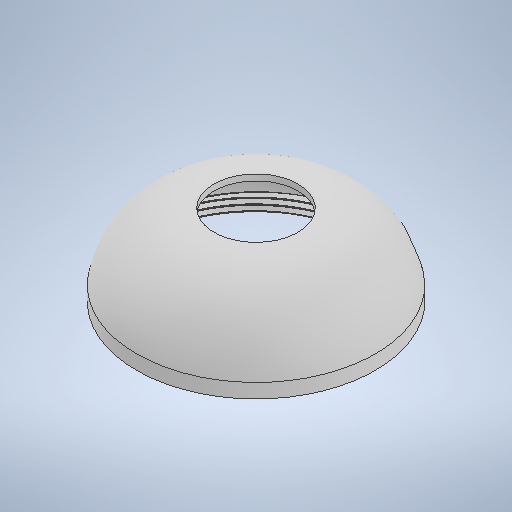
# Autodesk Inventor part: Cylinder Housing_cap
Saved by Autodesk Inventor 2025 (Build 290162000, 162)
## iProperties
Created: 2025-07-15
Part Number: Cylinder Housing_cap
Material: Generic
Document SubType Name: Modeling
Designer: mumin
Density: 1 g/cm^3
Appearance: Default
Author: mumin
Autodesk Inventor part; units mm, degrees
ref_plane "YZ Plane" through (0, 0, 0) normal (1, 0, 0) x (0, 1, 0)
ref_plane "XZ Plane" through (0, 0, 0) normal (0, 1, 0) x (-1, 0, 0)
ref_plane "XY Plane" through (0, 0, 0) normal (0, 0, 1) x (1, 0, 0)
sketch "Sketch1" plane through (0, 0, 0) normal (1, 0, 0) x (0, 1, 0)
  line L0 (-19.2867, 0) -> (115.7202, 0) projected
  line L1 (0, -116) -> (0, -121)
  line L2 (0, -116) -> (14.5, -116)
  line L3 (0, -121) -> (14.5, -121)
  line L4 (75.884, 0) -> (75.884, -42.5)
  arc A0 (14.5, -116) -> (75.884, -42.5) centre (1.1882, -42.5) ccw
  line L5 (75.884, -42.5) -> (82.0374, -42.5)
  arc A1 (14.5, -121) -> (82.0374, -42.5) centre (1.9607, -41.909) ccw
  point P0 (0, 0)
  dimension "d0" = 116
  dimension "d1" = 14.5
  dimension "d2" = 5
  dimension "d3" = 42.5
  constraints: 10 end point, 4 point on circle, 3 horizontal, 2 centre point, 2 vertical, 1 point on line, 1 tangent
  measures "d0" distance from line of L0 L1.start
  measures "d1" distance of L1.start L2.end
  measures "d2" distance of L1.start L1.end
  measures "d3" distance of L4.start L4.end
revolve "Revolution1" add sketch "Sketch1" angle 360 about axis through (0, -10, 0) along (0, 1, 0)
sketch "Sketch4" plane through (0, 0, 0) normal (0, 0, 1) x (1, 0, 0)
  arc A0 (74.226, 20) -> (32.226, 20) centre (53.226, 20) ccw
  line L0 (0, -8.9518) -> (0, 53.7108) projected
  line L1 (121, 0) -> (-121, 0) construction
  line L2 (32.226, 20) -> (32.226, 0)
  line L3 (32.226, 0) -> (74.226, 0)
  line L4 (74.226, 0) -> (74.226, 20)
  point P0 (0, 0)
  dimension "d26" = 42
  dimension "d27" = 53.226
  dimension "d28" = 20
  constraints: 6 end point, 2 point on circle, 1 centre point, 1 parallel, 1 point on line
  measures "d26" diameter of A0
  measures "d27" distance from line of L0 A0.centre
  measures "d28" distance from line of L1 A0.centre
extrude "LV Hole" cut sketch "Sketch4" against normal through all
thread "Thread2" size "M235x6" class "6H" standard "ANSI Metric M Profile" length 14.5
sketch "Sketch8" plane through (0, 14.5, 0) normal (1, 0, 0) x (0, 0, 1)
  line L0 (116, 0) -> (116, 14.5)
  line L1 (116, 14.5) -> (111.5512, 14.5)
  line L2 (111.5512, 14.5) -> (111.5512, 0)
  line L3 (111.5512, 0) -> (116, 0)
  line L4 (0, -83.9448) -> (0, 30.9075) projected
  constraints: 8 end point
revolve "Revolution4" add sketch "Sketch8" angle 360 about axis through (0, 14.5, 0) along (0, -1, 0) separate body
sketch "Sketch7" plane through (0, 14.5, 116) normal (-1, 0, 0) x (0, -1, 0)
  line L0 (-3.5001, -0.3036) -> (-3.0001, -0.3036) construction
  line L1 (0.4999, -4.1455) -> (-0.0001, -5.106) construction
  line L2 (-6.0001, -5.106) -> (-6.5001, -4.1455) construction
  line L3 (-2.5001, -0.3036) -> (-3.0001, 0.6569) construction
  line L4 (-3.0001, 0.6569) -> (-3.5001, -0.3036) construction
  line L5 (-6.0001, -5.106) -> (-5.5001, -4.1455) construction
  line L6 (-2.5001, -0.3036) -> (-0.5001, -4.1455)
  line L7 (-6.5001, -4.1455) -> (-5.5001, -4.1455) construction
  arc A0 (-6.5001, -4.1455) -> (-6.0001, -4.4489) centre (-6.0001, -3.8852) ccw construction
  line L8 (0.4999, -4.1455) -> (-0.5001, -4.1455) construction
  line L9 (-6.0001, -5.106) -> (-6.0001, -4.1455) construction
  line L10 (-0.0001, -5.106) -> (-0.0001, -4.1455) construction
  line L11 (-3.0001, 0.6569) -> (-3.0001, -0.0002) construction
  line L12 (-6.0001, -4.4489) -> (-0.0001, -4.4489)
  arc A1 (-6.0001, -4.4489) -> (-5.5001, -4.1455) centre (-6.0001, -3.8852) ccw
  line L13 (-0.5001, -4.1455) -> (-0.0001, -5.106) construction
  line L14 (-5.5001, -4.1455) -> (-3.5001, -0.3036)
  line L15 (-0.0001, -0.0002) -> (-0.0001, 0.0177)
  line L16 (-0.0001, 0.0177) -> (-0.0001, -0.0002)
  line L17 (-0.0001, -0.0002) -> (0.0334, -0.0002)
  arc A2 (-0.5001, -4.1455) -> (-0.0001, -4.4489) centre (-0.0001, -3.8852) ccw
  arc A3 (-0.0001, -4.4489) -> (0.4999, -4.1455) centre (-0.0001, -3.8852) ccw construction
  arc A4 (-3.0001, -0.0002) -> (-3.5001, -0.3036) centre (-3.0001, -0.5639) ccw
  arc A5 (-2.5001, -0.3036) -> (-3.0001, -0.0002) centre (-3.0001, -0.5639) ccw
  line L18 (-3.0001, -0.0002) -> (-3.0001, -0.3036) construction
  line L19 (-3.0001, -0.3036) -> (-2.5001, -0.3036) construction
  dimension "d51" = 55
  dimension "d52" = 0.9605
  dimension "d53" = 0.9605
  dimension "Sketch7_ThreadOffset" = 0
  dimension "Sketch7_MajorRadius" = 4.4488
  dimension "d56" = 6
  dimension "Sketch7_MinorRadius" = 0
  constraints: 40 end point, 12 point on circle, 10 parallel, 8 tangent, 6 centre point, 6 collinear, 2 midpoint, 2 point on line, 1 horizontal, 1 perpendicular, 3 other
  measures "d51" angle of L6 L14
  measures "d52" distance of L3.end L0.end
  measures "d53" distance of L1.end L10.end
  measures "Sketch7_ThreadOffset" distance between parallel lines of L15 L10
  measures "Sketch7_MajorRadius" distance from line of L12 L15.start
  measures "d56" distance from line of L1.end L9
  measures "Sketch7_MinorRadius" distance edge to line of A5 L17
coil "Coil3" sketch "Sketch7" operation cut axis through (0, 14.5, 0) along (0, -1, 0) pitch 6.006 turns 4.412254 hand right bodies 2
equation "\"d51\" = d58"
equation "\"d52\" = 0.160083 * Sketch7_Pitch"
equation "\"d53\" = 0.160083 * Sketch7_Pitch"
equation "\"d56\" = Sketch7_Pitch"
equation "\"d15\" = 55deg"
equation "\"Sketch2_Pitch\" = 8"
equation "\"d40\" = 55deg"
equation "\"Sketch5_Pitch\" = 6"
equation "\"d58\" = 55deg"
equation "\"Sketch7_Pitch\" = 6"
body "Solid1"
body "Solid4"
